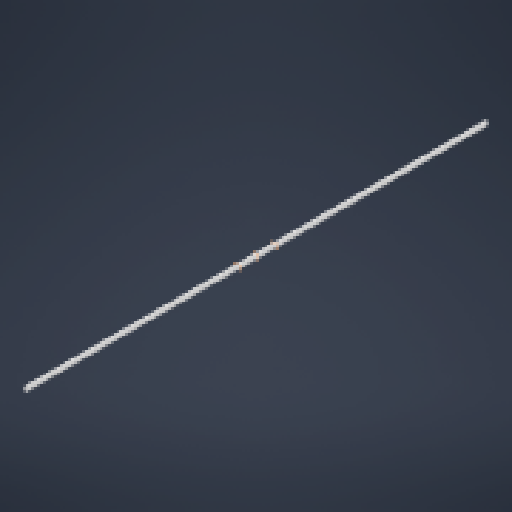
# Autodesk Inventor part: wingspar
Saved by Autodesk Inventor 2023 (Build 270158000, 158)
## iProperties
Created: 2022-12-27
Part Number: wingspar
Material: Generic
Document SubType Name: Modeling
Designer: Maciej
Density: 1 g/cm^3
Appearance: Default
Author: Maciej
Autodesk Inventor part; units mm, degrees
ref_plane "YZ Plane" through (0, 0, 0) normal (1, 0, 0) x (0, 1, 0)
ref_plane "XZ Plane" through (0, 0, 0) normal (0, 1, 0) x (-1, 0, 0)
ref_plane "XY Plane" through (0, 0, 0) normal (0, 0, 1) x (1, 0, 0)
sketch "Sketch1" plane through (0, 0, 0) normal (0, 0, 1) x (1, 0, 0)
  circle A0 centre (0, 0) radius 5
  circle A1 centre (0, 0) radius 4
  dimension "d0" = 10
  dimension "d1" = 8
  constraints: 2 centre point, 2 coincident
  measures "d0" diameter of A0
  measures "d1" diameter of A1
extrude "Extrusion1" add sketch "Sketch1" along normal blind 1000
ref_plane "Work Plane1" through (0, 0, 500) normal (0, 0, 1) x (1, 0, 0)
ref_plane "Work Plane2" through (0, 0, 540) normal (0, 0, 1) x (1, 0, 0)
ref_plane "Work Plane3" through (0, 0, 460) normal (0, 0, 1) x (1, 0, 0)
sketch "Sketch2" plane through (0, 0, 540) normal (0, 0, 1) x (1, 0, 0)
  circle A0 centre (0, 0) radius 4 projected
  circle A1 centre (0, 0) radius 5 projected
body "Solid1"
